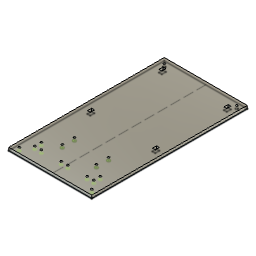
behavior_box_assembly (Autodesk Fusion 360 archive; units mm, degrees)
design "behavior_box_base"
part number: 2025-09-12-10-30-55-084
Autodesk Fusion 360 part; units mm, degrees
sketch "base_5mm_acrylic (1)" plane through (0, 0, 0) normal (0, 0, 1) x (1, 0, 0)
  line L0 (145.4499, -155.05) -> (145.4499, -162.9)
  line L1 (14.5499, -162.9003) -> (14.5499, -155.0503)
  line L2 (0, -300) -> (159.9999, -300)
  line L3 (139.9999, -24.7503) -> (139.9999, -16.9003)
  line L4 (19.9999, -155.0503) -> (19.9999, -162.9003)
  line L5 (14.5499, -16.9003) -> (19.9999, -16.9003)
  line L6 (14.5499, -24.7503) -> (14.5499, -16.9003)
  line L7 (159.9999, -300) -> (159.9999, 0)
  line L8 (19.9999, -162.9003) -> (14.5499, -162.9003)
  line L9 (139.9999, -155.05) -> (145.4499, -155.05)
  line L10 (19.9999, -24.7503) -> (14.5499, -24.7503)
  line L11 (14.5499, -155.0503) -> (19.9999, -155.0503)
  line L12 (139.9999, -16.9003) -> (145.4499, -16.9003)
  line L13 (145.4499, -16.9003) -> (145.4499, -24.7503)
  line L14 (145.4499, -24.7503) -> (139.9999, -24.7503)
  line L15 (0, 0) -> (0, -300)
  line L16 (139.9999, -162.9) -> (139.9999, -155.05)
  line L17 (159.9999, 0) -> (0, 0)
  line L18 (145.4499, -162.9) -> (139.9999, -162.9)
  line L19 (19.9999, -16.9003) -> (19.9999, -24.7503)
  spline S0 degree 3 poles (111.0098, -220.4076) (111.0098, -219.3031) (111.905, -218.4075) (113.0098, -218.4075) (114.1142, -218.4075) (115.0098, -219.3031) (115.0098, -220.4076) (115.0098, -221.5123) (114.1142, -222.4075) (113.0098, -222.4075) (111.905, -222.4075) (111.0098, -221.5123) (111.0098, -220.4076) knots 0 0 0 0 1 1 1 2 2 2 3 3 3 4 4 4 4
  spline S1 degree 3 poles (111.0098, -220.4076) (111.0098, -219.3031) (111.905, -218.4075) (113.0098, -218.4075) (114.1142, -218.4075) (115.0098, -219.3031) (115.0098, -220.4076) (115.0098, -221.5123) (114.1142, -222.4075) (113.0098, -222.4075) (111.905, -222.4075) (111.0098, -221.5123) (111.0098, -220.4076) knots 0 0 0 0 1 1 1 2 2 2 3 3 3 4 4 4 4
  spline S2 degree 3 poles (111.0098, -243.8604) (111.0098, -242.756) (111.905, -241.8605) (113.0098, -241.8605) (114.1142, -241.8605) (115.0098, -242.756) (115.0098, -243.8604) (115.0098, -244.9648) (114.1142, -245.8605) (113.0098, -245.8605) (111.905, -245.8605) (111.0098, -244.9648) (111.0098, -243.8604) knots 0 0 0 0 1 1 1 2 2 2 3 3 3 4 4 4 4
  spline S3 degree 3 poles (111.0098, -243.8604) (111.0098, -242.756) (111.905, -241.8605) (113.0098, -241.8605) (114.1142, -241.8605) (115.0098, -242.756) (115.0098, -243.8604) (115.0098, -244.9648) (114.1142, -245.8605) (113.0098, -245.8605) (111.905, -245.8605) (111.0098, -244.9648) (111.0098, -243.8604) knots 0 0 0 0 1 1 1 2 2 2 3 3 3 4 4 4 4
  spline S4 degree 3 poles (45.0121, -220.4076) (45.0121, -219.3031) (45.9075, -218.4075) (47.0121, -218.4075) (48.1166, -218.4075) (49.0121, -219.3031) (49.0121, -220.4076) (49.0121, -221.5123) (48.1166, -222.4075) (47.0121, -222.4075) (45.9075, -222.4075) (45.0121, -221.5123) (45.0121, -220.4076) knots 0 0 0 0 1 1 1 2 2 2 3 3 3 4 4 4 4
  spline S5 degree 3 poles (45.0121, -220.4076) (45.0121, -219.3031) (45.9075, -218.4075) (47.0121, -218.4075) (48.1166, -218.4075) (49.0121, -219.3031) (49.0121, -220.4076) (49.0121, -221.5123) (48.1166, -222.4075) (47.0121, -222.4075) (45.9075, -222.4075) (45.0121, -221.5123) (45.0121, -220.4076) knots 0 0 0 0 1 1 1 2 2 2 3 3 3 4 4 4 4
  spline S6 degree 3 poles (45.0121, -243.8604) (45.0121, -242.756) (45.9075, -241.8605) (47.0121, -241.8605) (48.1166, -241.8605) (49.0121, -242.756) (49.0121, -243.8604) (49.0121, -244.9648) (48.1166, -245.8605) (47.0121, -245.8605) (45.9075, -245.8605) (45.0121, -244.9648) (45.0121, -243.8604) knots 0 0 0 0 1 1 1 2 2 2 3 3 3 4 4 4 4
  spline S7 degree 3 poles (45.0121, -243.8604) (45.0121, -242.756) (45.9075, -241.8605) (47.0121, -241.8605) (48.1166, -241.8605) (49.0121, -242.756) (49.0121, -243.8604) (49.0121, -244.9648) (48.1166, -245.8605) (47.0121, -245.8605) (45.9075, -245.8605) (45.0121, -244.9648) (45.0121, -243.8604) knots 0 0 0 0 1 1 1 2 2 2 3 3 3 4 4 4 4
  spline S8 degree 3 poles (134.8502, -272.9937) (134.8502, -271.8892) (135.7454, -270.9937) (136.8502, -270.9937) (137.9546, -270.9937) (138.8502, -271.8892) (138.8502, -272.9937) (138.8502, -274.0981) (137.9546, -274.9937) (136.8502, -274.9937) (135.7454, -274.9937) (134.8502, -274.0981) (134.8502, -272.9937) knots 0 0 0 0 1 1 1 2 2 2 3 3 3 4 4 4 4
  spline S9 degree 3 poles (84.8501, -272.9937) (84.8501, -271.8892) (85.7457, -270.9937) (86.8501, -270.9937) (87.9546, -270.9937) (88.8501, -271.8892) (88.8501, -272.9937) (88.8501, -274.0981) (87.9546, -274.9937) (86.8501, -274.9937) (85.7457, -274.9937) (84.8501, -274.0981) (84.8501, -272.9937) knots 0 0 0 0 1 1 1 2 2 2 3 3 3 4 4 4 4
  spline S10 degree 3 poles (33.8503, -272.9937) (33.8503, -271.8892) (34.7457, -270.9937) (35.8503, -270.9937) (36.9549, -270.9937) (37.8503, -271.8892) (37.8503, -272.9937) (37.8503, -274.0981) (36.9549, -274.9937) (35.8503, -274.9937) (34.7457, -274.9937) (33.8503, -274.0981) (33.8503, -272.9937) knots 0 0 0 0 1 1 1 2 2 2 3 3 3 4 4 4 4
  spline S11 degree 3 poles (122.1502, -272.9937) (122.1502, -271.8892) (123.0454, -270.9937) (124.1502, -270.9937) (125.2546, -270.9937) (126.1502, -271.8892) (126.1502, -272.9937) (126.1502, -274.0981) (125.2546, -274.9937) (124.1502, -274.9937) (123.0454, -274.9937) (122.1502, -274.0981) (122.1502, -272.9937) knots 0 0 0 0 1 1 1 2 2 2 3 3 3 4 4 4 4
  spline S12 degree 3 poles (134.8502, -260.294) (134.8502, -259.1896) (135.7454, -258.294) (136.8502, -258.294) (137.9546, -258.294) (138.8502, -259.1896) (138.8502, -260.294) (138.8502, -261.3984) (137.9546, -262.294) (136.8502, -262.294) (135.7454, -262.294) (134.8502, -261.3984) (134.8502, -260.294) knots 0 0 0 0 1 1 1 2 2 2 3 3 3 4 4 4 4
  spline S13 degree 3 poles (72.1501, -272.9937) (72.1501, -271.8892) (73.0457, -270.9937) (74.1501, -270.9937) (75.2546, -270.9937) (76.1501, -271.8892) (76.1501, -272.9937) (76.1501, -274.0981) (75.2546, -274.9937) (74.1501, -274.9937) (73.0457, -274.9937) (72.1501, -274.0981) (72.1501, -272.9937) knots 0 0 0 0 1 1 1 2 2 2 3 3 3 4 4 4 4
  spline S14 degree 3 poles (21.1503, -272.9937) (21.1503, -271.8892) (22.0457, -270.9937) (23.1503, -270.9937) (24.2549, -270.9937) (25.1503, -271.8892) (25.1503, -272.9937) (25.1503, -274.0981) (24.2549, -274.9937) (23.1503, -274.9937) (22.0457, -274.9937) (21.1503, -274.0981) (21.1503, -272.9937) knots 0 0 0 0 1 1 1 2 2 2 3 3 3 4 4 4 4
  spline S15 degree 3 poles (21.1503, -260.294) (21.1503, -259.1896) (22.0457, -258.294) (23.1503, -258.294) (24.2549, -258.294) (25.1503, -259.1896) (25.1503, -260.294) (25.1503, -261.3984) (24.2549, -262.294) (23.1503, -262.294) (22.0457, -262.294) (21.1503, -261.3984) (21.1503, -260.294) knots 0 0 0 0 1 1 1 2 2 2 3 3 3 4 4 4 4
  spline S16 degree 3 poles (12.0002, -289.9998) (12.0002, -291.1044) (11.1048, -291.9998) (10.0002, -291.9998) (8.8957, -291.9998) (8.0002, -291.1044) (8.0002, -289.9998) (8.0002, -288.8952) (8.8957, -287.9998) (10.0002, -287.9998) (11.1048, -287.9998) (12.0002, -288.8952) (12.0002, -289.9998) knots 0 0 0 0 1 1 1 2 2 2 3 3 3 4 4 4 4
  spline S17 degree 3 poles (152.0002, -289.9998) (152.0002, -291.1044) (151.1048, -291.9998) (150.0002, -291.9998) (148.8957, -291.9998) (148.0002, -291.1044) (148.0002, -289.9998) (148.0002, -288.8952) (148.8957, -287.9998) (150.0002, -287.9998) (151.1048, -287.9998) (152.0002, -288.8952) (152.0002, -289.9998) knots 0 0 0 0 1 1 1 2 2 2 3 3 3 4 4 4 4
  spline S18 degree 3 poles (11.9999, -10) (11.9999, -11.1045) (11.1045, -12) (9.9999, -12) (8.8954, -12) (7.9999, -11.1045) (7.9999, -10) (7.9999, -8.8954) (8.8954, -8) (9.9999, -8) (11.1045, -8) (11.9999, -8.8954) (11.9999, -10) knots 0 0 0 0 1 1 1 2 2 2 3 3 3 4 4 4 4
  spline S19 degree 3 poles (151.9999, -10) (151.9999, -11.1045) (151.1045, -12) (149.9999, -12) (148.8954, -12) (147.9999, -11.1045) (147.9999, -10) (147.9999, -8.8954) (148.8954, -8) (149.9999, -8) (151.1045, -8) (151.9999, -8.8954) (151.9999, -10) knots 0 0 0 0 1 1 1 2 2 2 3 3 3 4 4 4 4
  line L20 (79.9999, 0) -> (79.9999, -300) construction
  point P0 (10, -287.9998)
  dimension "d37" = 159.9999
  dimension "d38" = 300
  dimension "d42" = 120
  dimension "d43" = 120
  dimension "d44" = 5.45
  dimension "d47" = 19.9999
  dimension "d51" = 12.0002
  dimension "d52" = 12.0002
  dimension "d54" = 10
  dimension "d55" = 11.9999
  dimension "d56" = 10
  dimension "d57" = 7.9999
  dimension "d60" = 146
  dimension "d61" = 145.9997
  dimension "d62" = 130.9
  dimension "d70" = 7.85
  dimension "d73" = 16.9003
  dimension "d74" = 16.9003
  dimension "d71" = 130.3
  constraint perpendicular L15 L17
  constraint perpendicular L7 L17
  constraint perpendicular L2 L7
  constraint coincident L15.start L17.end
  constraint horizontal L17
  constraint equal L8 L11
  constraint equal L11 L18
  constraint equal L9 L18
  constraint equal L9 L14
  constraint equal L12 L14
  constraint equal L10 L12
  constraint equal L5 L10
  constraint coincident S16 P0
  constraint coincident L17 L20.start
  constraint perpendicular L17 L20
  constraint midpoint L2 L20.end
  constraint symmetric L6 L13 L20
  constraint equal L6 L19
  constraint equal L3 L19
  constraint equal L3 L13
  constraint equal L0 L13
  constraint equal L0 L16
  constraint equal L4 L16
  constraint equal L1 L4
  measures "d37" distance of L7.end L15.start
  measures "d38" distance of L2 L17
  measures "d42" distance of L4 L16
  measures "d43" distance of L3 L19
  measures "d44" distance of L1 L4
  measures "d47" distance of L3 L7
  measures "d51" distance of L15 S16.start
  measures "d52" distance of L2 P0
  measures "d54" distance of L17 S18.start
  measures "d55" distance of L15 S18.start
  measures "d56" distance of L17 S19.start
  measures "d57" distance of L7 S19.start
  measures "d60" distance of L5 L8
  measures "d61" distance of L12 L18
  measures "d62" distance of L0 L1
  measures "d70" distance of L4.start L4.end
  measures "d73" distance of L5 L17
  measures "d74" distance of L12 L17
extrude "Extrude1" add sketch "base_5mm_acrylic (1)" along normal blind 5.6
extrude "Extrude3" [suppressed]
extrude "Extrude2" [suppressed]
equation "acr_thickness = 5.6 mm" comment "thickness of acrylic used to laser cut parts"
equation "kerf = 0.15 mm"
equation "d7 = acr_thickness"
equation "d31 = acr_thickness"
equation "d44 = acr_thickness - 1 * kerf"
equation "d58 = -acr_thickness"
equation "d70 = 8.00 mm - 1 * kerf"
named bodies: "Base"

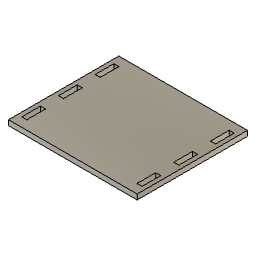
design "behavior_box_top_closed" references "behavior_box_base"
part number: 2025-09-14-13-40-32-552
Autodesk Fusion 360 part; units mm, degrees
sketch "Sketch1" plane through (0, 0, 0) normal (0, 0, 1) x (1, 0, 0)
  line L0 (135.4499, -70.1501) -> (129.9999, -70.1501)
  line L1 (135.4499, -49.8502) -> (135.4499, -70.1501)
  line L2 (135.4499, -30.1501) -> (129.9999, -30.1501)
  line L3 (0, -119.9999) -> (0, 0)
  line L4 (129.9999, -9.8499) -> (135.4499, -9.8499)
  line L5 (135.4499, -9.8499) -> (135.4499, -30.1501)
  line L6 (4.5499, -89.8142) -> (9.9999, -89.8142)
  line L7 (9.9999, -89.8142) -> (9.9999, -110.1141)
  line L8 (129.9999, -49.8502) -> (135.4499, -49.8502)
  line L9 (129.9999, -89.8486) -> (135.4499, -89.8486)
  line L10 (9.9999, -49.8499) -> (9.9999, -70.1497)
  line L11 (9.9999, -110.1141) -> (4.5499, -110.1141)
  line L12 (129.9999, -70.1501) -> (129.9999, -49.8502)
  line L13 (139.9999, 0) -> (139.9999, -119.9999)
  line L14 (9.9999, -9.8504) -> (9.9999, -30.1501)
  line L15 (9.9999, -70.1497) -> (4.5499, -70.1498)
  line L16 (4.5499, -70.1498) -> (4.5499, -49.8499)
  line L17 (4.5499, -30.1501) -> (4.5499, -9.8504)
  line L18 (129.9999, -110.1485) -> (129.9999, -89.8486)
  line L19 (129.9999, -30.1501) -> (129.9999, -9.8499)
  line L20 (4.5499, -110.1141) -> (4.5499, -89.8142)
  line L21 (9.9999, -30.1501) -> (4.5499, -30.1501)
  line L22 (139.9999, -119.9999) -> (0, -119.9999)
  line L23 (4.5499, -9.8504) -> (9.9999, -9.8504)
  line L24 (0, 0) -> (139.9999, 0)
  line L25 (135.4499, -110.1485) -> (129.9999, -110.1485)
  line L26 (135.4499, -89.8486) -> (135.4499, -110.1485)
  line L27 (4.5499, -49.8499) -> (9.9999, -49.8499)
  line L28 (69.9999, 0) -> (69.9999, -119.9999) construction
  dimension "d1" = 5.45
  dimension "d2" = 119.9999
  dimension "d3" = 139.9999
  dimension "d5" = 120
  constraint vertical L13
  constraint horizontal L24
  constraint midpoint L24 L28.start
  constraint midpoint L22 L28.end
  constraint collinear L16 L17
  constraint collinear L16 L20
  constraint collinear L12 L19
  constraint collinear L12 L18
  constraint collinear L2 L21
  constraint coincident L3.end L24.start
  constraint perpendicular L14 L23
  constraint perpendicular L17 L21
  constraint perpendicular L16 L27
  constraint perpendicular L15 L16
  constraint perpendicular L6 L20
  constraint perpendicular L11 L20
  constraint perpendicular L9 L26
  constraint perpendicular L25 L26
  constraint perpendicular L0 L1
  constraint perpendicular L1 L8
  constraint perpendicular L8 L12
  constraint perpendicular L4 L19
  constraint perpendicular L4 L5
  constraint equal L4 L23
  constraint collinear L1 L5
  constraint collinear L1 L26
  measures "d1" distance of L14 L17
  measures "d2" distance of L22 L24
  measures "d3" distance of L3 L13
  measures "d5" distance of L7 L18
other "Derived from behavior_box_base"
extrude "Extrude1" add sketch "Sketch1" along normal blind 5.6
equation "d1 = acr_thickness_Ref - kerf_Ref"
equation "acr_thickness_Ref = 5.6 mm" comment "thickness of acrylic used to laser cut parts"
equation "kerf_Ref = 0.15 mm"
equation "d8 = acr_thickness_Ref"

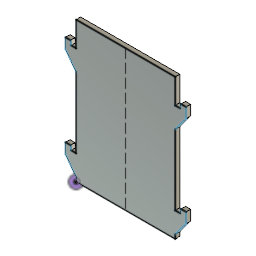
design "behavior_box_front" references "behavior_box_base"
part number: 2025-09-12-13-42-14-660
Autodesk Fusion 360 part; units mm, degrees
sketch "Sketch1" plane through (0, 0, 0) normal (0, 1, 0) x (1, 0, 0)
sketch "Sketch2" plane through (0, 0, 0) normal (0, 1, 0) x (1, 0, 0)
  line L0 (0, -115.0743) -> (0, -30.0003)
  line L1 (-12.9995, -144.9995) -> (-12.9995, -132.5621)
  line L2 (-12.9995, -132.5621) -> (0, -115.0743)
  line L3 (120.0003, 0) -> (120.0003, -5.0002)
  line L4 (0, -5.0002) -> (0, 0)
  line L5 (120.0003, -5.0002) -> (119.9999, -5.0002)
  line L6 (-6.7911, -35.0005) -> (-12.9995, -35.0005)
  line L7 (0, -30.0003) -> (-5.795, -30.0003)
  line L8 (0, 0) -> (120.0003, 0)
  line L9 (120.0003, -115.0661) -> (120.0121, -115.0661)
  line L10 (-12.9995, -22.5003) -> (0, -5.0002)
  line L11 (126.8044, -144.9995) -> (125.7953, -139.9993)
  line L12 (120.0008, -29.9993) -> (120.0003, -29.9993)
  line L13 (120.0121, -115.0661) -> (133.0007, -132.5621)
  line L14 (126.8455, -35.0005) -> (125.7953, -29.9993)
  line L15 (120.0003, -29.9993) -> (120.0003, -115.0661)
  line L16 (133.0007, -132.5621) -> (133.0007, -144.9995)
  line L17 (120.0006, -139.9993) -> (120.0003, -139.9993)
  line L18 (-12.9995, -35.0005) -> (-12.9995, -22.5003)
  line L19 (133.0007, -144.9995) -> (126.8044, -144.9995)
  line L20 (-5.795, -30.0003) -> (-6.7911, -35.0005)
  line L21 (133.0007, -22.5003) -> (133.0007, -35.0005)
  line L22 (133.0007, -35.0005) -> (126.8455, -35.0005)
  line L23 (119.9999, -5.0002) -> (133.0007, -22.5003)
  line L24 (0, -169.9998) -> (0, -139.9993)
  line L25 (120.0003, -139.9993) -> (120.0003, -169.9998)
  line L26 (0, -139.9993) -> (-5.795, -139.9993)
  line L27 (120.0003, -169.9998) -> (0, -169.9998)
  line L28 (-6.8033, -144.9995) -> (-12.9995, -144.9995)
  line L29 (-5.795, -139.9993) -> (-6.8033, -144.9995)
  line L30 (120.0003, -139.9993) -> (125.7953, -139.9993)
  line L31 (120.0003, -29.9993) -> (125.7953, -29.9993)
  line L32 (60.0001, -169.9998) -> (60.0001, 0) construction
  dimension "d1" = 120.0003
  dimension "d2" = 169.9998
  dimension "d4" = 30.0006
  dimension "d5" = 5.0002
  dimension "d7" = 5.0002
  dimension "d8" = 5.795
  dimension "d9" = 12.5002
  dimension "d11" = 35.0005
  dimension "d12" = 5.0002
  dimension "d16" = 5.795
  dimension "d18" = 5.795
  dimension "d19" = 5.795
  dimension "d22" = 30.0006
  dimension "d28" = 110
  dimension "d29" = 146.0002
  constraint perpendicular L24 L27
  constraint perpendicular L25 L27
  constraint perpendicular L8 L15
  constraint perpendicular L0 L8
  constraint perpendicular L0 L7
  constraint collinear L6 L22
  constraint collinear L0 L4
  constraint collinear L3 L15
  constraint collinear L0 L24
  constraint collinear L15 L25
  constraint collinear L19 L28
  constraint collinear L1 L18
  constraint collinear L16 L21
  constraint coincident L4.end L8.start
  constraint horizontal L8
  constraint equal L18 L21
  constraint equal L1 L16
  constraint equal L3 L4
  constraint equal L24 L25
  constraint equal L2 L13
  constraint perpendicular L25 L30
  constraint perpendicular L15 L31
  constraint equal L7 L31
  constraint equal L30 L31
  constraint equal L26 L30
  constraint equal L19 L28
  constraint midpoint L27 L32.start
  constraint midpoint L8 L32.end
  constraint symmetric L26 L30 L32
  constraint vertical L16
  measures "d1" distance of L0 L15
  measures "d2" distance of L8 L27
  measures "d4" distance of L24.start L24.end
  measures "d5" distance of L6 L7
  measures "d7" distance of L26 L28
  measures "d8" distance of L0.end L7.end
  measures "d9" distance of L6.end L10.start
  measures "d11" distance of L6 L8
  measures "d12" distance of L4.start L4.end
  measures "d16" distance of L24.end L26.end
  measures "d18" distance of L11.end L17.end
  measures "d19" distance of L14.end L12.end
  measures "d22" distance of L27 L30
  measures "d28" distance of L30 L31
  measures "d29" distance of L1 L16
other "Derived from behavior_box_base"
extrude "Extrude1" add sketch "Sketch2" along normal blind 5.6
equation "d8 = acr_thickness_Ref + 1.3 * kerf_Ref"
equation "acr_thickness_Ref = 5.6 mm" comment "thickness of acrylic used to laser cut parts"
equation "kerf_Ref = 0.15 mm"
equation "d25 = acr_thickness_Ref"

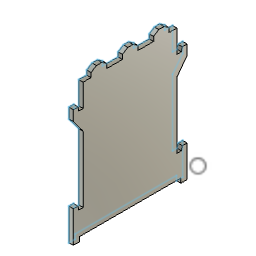
design "behavior_box_side" references "behavior_box_base"
part number: 2025-09-12-13-15-45-641
Autodesk Fusion 360 part; units mm, degrees
sketch "Sketch3" plane through (0, 0, 0) normal (1, 0, 0) x (0, 1, 0)
  line L0 (-19.607, 134.9148) -> (-32.6169, 118.167)
  line L1 (-19.607, 38.2007) -> (-19.607, -2.5486)
  line L2 (-102.5423, 172.4703) -> (-102.5423, 178.0703)
  line L3 (-42.7124, 178.0703) -> (-42.7124, 172.4703)
  line L4 (-129.016, 182.4513) -> (-122.5425, 178.0703)
  line L5 (-136.0157, 182.4513) -> (-129.016, 182.4513)
  line L6 (-49.1979, 182.4513) -> (-42.7124, 178.0703)
  line L7 (-25.8097, 148.1999) -> (-19.607, 148.1999)
  line L8 (-95.6509, 182.4513) -> (-89.0008, 182.4513)
  line L9 (-26.8139, 143.2014) -> (-25.8097, 148.1999)
  line L10 (-157.6068, 3.2014) -> (-157.6068, -2.5486)
  line L11 (-32.6089, 143.2014) -> (-26.8139, 143.2014)
  line L12 (-142.8034, 178.0703) -> (-136.0157, 182.4513)
  line L13 (-27.6069, 3.2014) -> (-157.6068, 3.2014)
  line L14 (-19.607, 148.1999) -> (-19.607, 134.9148)
  line L15 (-32.6089, 172.4703) -> (-32.6089, 143.2014)
  line L16 (-102.5423, 178.0703) -> (-95.6509, 182.4513)
  line L17 (-26.8219, 33.2014) -> (-25.562, 38.2007)
  line L18 (-82.5216, 178.0703) -> (-82.5216, 172.4703)
  line L19 (-142.8034, 172.4703) -> (-142.8034, 178.0703)
  line L20 (-42.7124, 172.4703) -> (-32.6089, 172.4703)
  line L21 (-55.9472, 182.4513) -> (-49.1979, 182.4513)
  line L22 (-82.5216, 172.4703) -> (-62.5214, 172.4703)
  line L23 (-122.5425, 172.4703) -> (-102.5423, 172.4703)
  line L24 (-152.9069, 172.4703) -> (-142.8034, 172.4703)
  line L25 (-32.6169, 118.167) -> (-32.6169, 33.2014)
  line L26 (-159.4042, 148.1999) -> (-158.7019, 143.2014)
  line L27 (-122.5425, 178.0703) -> (-122.5425, 172.4703)
  line L28 (-159.6519, 38.2007) -> (-158.7119, 33.2014)
  line L29 (-25.562, 38.2007) -> (-19.607, 38.2007)
  line L30 (-62.5214, 172.4703) -> (-62.5214, 178.0703)
  line L31 (-152.9169, 33.2014) -> (-158.7119, 33.2014)
  line L32 (-89.0008, 182.4513) -> (-82.5216, 178.0703)
  line L33 (-62.5214, 178.0703) -> (-55.9472, 182.4513)
  line L34 (-158.7019, 143.2014) -> (-152.9069, 143.2014)
  line L35 (-152.9169, 33.2014) -> (-152.9169, 118.0218)
  line L36 (-152.9069, 143.2014) -> (-152.9069, 172.4703)
  line L37 (-165.6069, 38.2007) -> (-159.6519, 38.2007)
  line L38 (-32.6169, 33.2014) -> (-26.8219, 33.2014)
  line L39 (-152.9169, 118.0218) -> (-165.6069, 135.069)
  line L40 (-27.6069, -2.5486) -> (-27.6069, 3.2014)
  line L41 (-19.607, -2.5486) -> (-27.6069, -2.5486)
  line L42 (-165.6069, 135.069) -> (-165.6069, 148.1999)
  line L43 (-157.6068, -2.5486) -> (-165.6069, -2.5486)
  line L44 (-165.6069, 148.1999) -> (-159.4042, 148.1999)
  line L45 (-165.6069, -2.5486) -> (-165.6069, 38.2007)
  dimension "d1" = 20.0002
  dimension "d2" = 7.9998
  dimension "d3" = 8
  dimension "d4" = 145.9999
  dimension "d5" = 5.795
  dimension "d6" = 120.3
  dimension "d11" = 5.795
  dimension "d12" = 4.9993
  dimension "d13" = 4.9993
  dimension "d14" = 4.9985
  dimension "d15" = 4.9985
  dimension "d16" = 5.795
  dimension "d23" = 5.75
  dimension "d25" = 184.9999
  dimension "d26" = 169.2689
  dimension "d27" = 29.2689
  dimension "d28" = 30
  dimension "d29" = 130
  dimension "d30" = 110
  dimension "d31" = 5.6
  dimension "d32" = 120.2981
  constraint perpendicular L15 L20
  constraint perpendicular L24 L36
  constraint perpendicular L34 L36
  constraint perpendicular L42 L44
  constraint perpendicular L31 L35
  constraint perpendicular L37 L45
  constraint perpendicular L43 L45
  constraint perpendicular L10 L43
  constraint perpendicular L10 L13
  constraint perpendicular L13 L40
  constraint perpendicular L40 L41
  constraint perpendicular L1 L41
  constraint perpendicular L1 L29
  constraint perpendicular L25 L38
  constraint perpendicular L7 L14
  constraint perpendicular L11 L15
  constraint equal L22 L23
  constraint collinear L1 L14
  constraint collinear L42 L45
  constraint collinear L8 L21
  constraint collinear L5 L8
  constraint collinear L20 L22
  constraint collinear L22 L23
  constraint collinear L23 L24
  constraint equal L20 L24
  constraint equal L15 L36
  constraint equal L11 L34
  constraint equal L31 L34
  constraint equal L31 L38
  constraint parallel L29 L38
  constraint equal L29 L37
  constraint equal L7 L44
  constraint collinear L29 L37
  constraint collinear L31 L38
  constraint collinear L7 L44
  constraint equal L10 L40
  constraint vertical L19
  constraint vertical L27
  constraint vertical L2
  constraint vertical L18
  constraint vertical L30
  constraint vertical L3
  constraint equal L19 L27
  constraint equal L2 L27
  constraint equal L2 L18
  constraint equal L18 L30
  constraint equal L3 L30
  constraint vertical L36
  measures "d1" distance of L18.end L22.end
  measures "d2" distance of L1.end L40.start
  measures "d3" distance of L10.end L43.end
  measures "d4" distance of L1 L45
  measures "d5" distance of L17.start L25.end
  measures "d6" distance of L25 L35
  measures "d11" distance of L34.end L26.end
  measures "d12" distance of L29 L38
  measures "d13" distance of L31 L37
  measures "d14" distance of L7 L11
  measures "d15" distance of L34 L44
  measures "d16" distance of L11.start L9.start
  measures "d23" distance of L10.end L10.start
  measures "d25" distance of L5 L43
  measures "d26" distance of L13 L23
  measures "d27" distance of L24 L34
  measures "d28" distance of L13 L31
  measures "d29" distance of L10 L40
  measures "d30" distance of L31 L34
  measures "d31" distance of L4.end L23.start
  measures "d32" distance of L15 L36
other "Derived from behavior_box_base"
extrude "Extrude1" add sketch "Sketch3" along normal blind 5.6
extrude "Extrude2" [rolled back] along distance 5.6 taper angle 0
equation "d5 = acr_thickness_Ref + 1.3 * kerf_Ref"
equation "d6 = 120 mm + 2 * kerf_Ref"
equation "acr_thickness_Ref = 5.6 mm" comment "thickness of acrylic used to laser cut parts"
equation "kerf_Ref = 0.15 mm"
equation "d19 = acr_thickness_Ref"
equation "d21 = acr_thickness_Ref"
equation "d23 = acr_thickness_Ref + kerf_Ref"
equation "d31 = acr_thickness_Ref"
